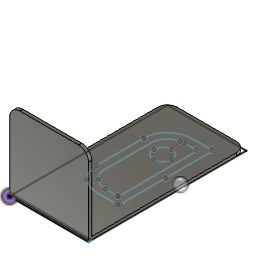
Switch Left Bookend (Autodesk Fusion 360 design; units mm, degrees)
Autodesk Fusion 360 part; units mm, degrees
note: some values were not read from the file. Chosen so that the rebuilt part matches the saved one: which pieces of a blend or face edit are solid.
sketch "Sketch1" plane through (0, 0, 0) normal (0, 0, 1) x (1, 0, 0)
  line L0 (0, 0) -> (50, 0)
  line L1 (50, 0) -> (50, 100)
  line L2 (50, 100) -> (0, 100)
  line L3 (0, 100) -> (0, 0)
  line L4 (0, 0) -> (50, 0)
  line L5 (50, 0) -> (50, 2)
  line L6 (50, 2) -> (0, 2)
  line L7 (0, 2) -> (0, 0)
  line L8 (34.5636, 34.4661) -> (34.5636, 84.5568)
  line L9 (34.5636, 84.5568) -> (33.9119, 84.5568)
  spline S0 degree 3 poles (33.9119, 84.5568) (31.3963, 84.5567) (28.8804, 84.5751) (26.365, 84.5464) knots 2 2 2 2 3 3 3 3
  ellipse E0 centre (47.6158, 60.5322) end of major axis (76.3213, 39.5009) minor radius 14.3732 (26.365, 84.5464) -> (23.8572, 84.3209) ccw
  spline S1 degree 3 poles (23.8572, 84.3209) (19.1392, 83.4681) (15.4509, 79.0364) (15.4484, 74.2383) (15.4432, 64.3821) (15.418, 54.5257) (15.4644, 44.6697) (15.4782, 41.7272) (16.6921, 39.2323) (18.8504, 37.224) knots 4 4 4 4 5 5 5 6 6 6 7 7 7 7
  spline S2 degree 3 poles (18.8504, 37.224) (20.9228, 35.2959) (23.4181, 34.4467) (26.2187, 34.4355) knots 7 7 7 7 8 8 8 8
  spline S3 degree 3 poles (26.2187, 34.4355) (28.8282, 34.4249) (31.4379, 34.4327) (34.0474, 34.4345) knots 8 8 8 8 9 9 9 9
  spline S4 degree 3 poles (34.0474, 34.4345) (34.2116, 34.4346) (34.3757, 34.454) (34.5636, 34.4661) knots 9 9 9 9 10 10 10 10
  spline S5 degree 3 poles (39.447, 59.4869) (39.447, 49.797) (39.447, 40.107) (39.4468, 30.4169) knots 0 0 0 0 1 1 1 1
  spline S6 degree 3 poles (39.4468, 30.4169) (39.4468, 29.6608) (39.3671, 29.5827) (38.611, 29.5829) knots 1 1 1 1 2 2 2 2
  spline S7 degree 3 poles (38.611, 29.5829) (34.4982, 29.5843) (30.3857, 29.5861) (26.2732, 29.5868) (22.066, 29.5875) (18.382, 30.9667) (15.3248, 33.8662) knots 2 2 2 2 3 3 3 4 4 4 4
  ellipse E1 centre (94.1785, 83.9771) end of major axis (175.7393, 130.6607) minor radius 36.8762 (10.9507, 41.7409) -> (15.3248, 33.8662) ccw
  spline S8 degree 3 poles (10.9507, 41.7409) (10.766, 42.6338) (10.6197, 43.5543) (10.6175, 44.4625) knots 5 5 5 5 6 6 6 6
  spline S9 degree 3 poles (10.6175, 44.4625) (10.5946, 54.4717) (10.465, 64.4835) (10.6545, 74.4892) knots 6 6 6 6 7 7 7 7
  spline S10 degree 3 poles (10.6545, 74.4892) (10.7735, 80.7614) (13.9901, 85.298) (19.6506, 88.0297) (21.7359, 89.036) (23.9778, 89.4054) (26.2894, 89.3998) (30.3831, 89.3897) (34.477, 89.3984) (38.5708, 89.3992) knots 7 7 7 7 8 8 8 9 9 9 10 10 10 10
  spline S11 degree 3 poles (38.5708, 89.3992) (39.4186, 89.3993) (39.447, 89.3705) (39.447, 88.5007) (39.447, 78.8293) (39.447, 69.1582) (39.447, 59.4869) knots 10 10 10 10 11 11 11 12 12 12 12
  spline S12 degree 3 poles (19.9368, 71.4906) (19.8468, 74.4011) (22.2958, 77.0965) (25.5212, 77.0856) knots 0 0 0 0 1 1 1 1
  spline S13 degree 3 poles (25.5212, 77.0856) (28.6661, 77.0751) (31.1925, 74.7102) (31.1724, 71.3632) knots 1 1 1 1 2 2 2 2
  spline S14 degree 3 poles (31.1724, 71.3632) (31.1523, 68.0382) (28.3565, 65.7588) (25.4577, 65.8303) knots 2 2 2 2 3 3 3 3
  spline S15 degree 3 poles (25.4577, 65.8303) (22.3345, 65.9072) (19.9164, 68.3391) (19.9368, 71.4906) knots 3 3 3 3 4 4 4 4
  dimension "d1" = 50
  dimension "d2" = 100
  dimension "d3" = 2
  constraint horizontal L0
  constraint vertical L1
  constraint horizontal L2
  constraint vertical L3
  constraint coincident L0.start L3.end
  constraint horizontal L4
  constraint vertical L5
  constraint horizontal L6
  constraint vertical L7
  measures "d1" distance of L0.start L0.end
  measures "d2" distance of L0.start L2.end
  measures "d3" distance of L0.start L6.end
extrude "Extrude1" add sketch "Sketch1" along normal blind 2 contours L1 L2 L3 L6 | L8 L9 S0 E0 S1 S2 S3 S4 | S5 S6 S7 E1 S8 S9 S10 S11 | S12 S13 S14 S15
extrude "Extrude2" cut sketch "Sketch1" along normal blind 1 contours S5 S6 S7 E1 S8 S9 S10 S11 | S12 S13 S14 S15
extrude "Extrude3" add sketch "Sketch1" along normal blind 50 contours L0 L1 L3 L4 L5 L6 L7
fillet "Fillet1" radius 6.25 2 edges at (0, 100, 1) (50, 100, 1)
fillet "Fillet2" radius 6.25 2 edges at (0, 1, 50) (50, 1, 50)
fillet "Fillet3" radius 1 1 edges at (25, 0, 0)
